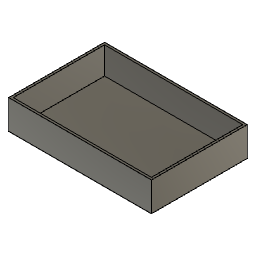
Container v1 (Autodesk Fusion 360 design; units mm, degrees)
Autodesk Fusion 360 part; units mm, degrees
sketch "Sketch1" plane through (0, 0, 0) normal (0, 0, 1) x (1, 0, 0)
  line L0 (63.38, 42.565) -> (-63.38, 42.565)
  line L1 (-63.38, 42.565) -> (-63.38, -42.565)
  line L2 (-63.38, -42.565) -> (63.38, -42.565)
  line L3 (63.38, -42.565) -> (63.38, 42.565)
  line L4 (63.38, 42.565) -> (-63.38, -42.565) construction
  line L5 (-63.38, 42.565) -> (63.38, -42.565) construction
  dimension "d1" = 126.76
  dimension "d2" = 85.13
  constraint horizontal L0
  constraint perpendicular L0 L1
  constraint parallel L0 L2
  constraint parallel L1 L3
  constraint coincident L4 origin
  constraint coincident L5 origin
  measures "d1" distance of L1.end L2.end
  measures "d2" distance of L0.end L1.end
extrude "Extrude1" add sketch "Sketch1" along normal blind 26
shell "Shell1" thickness 2 removed faces 1 at (21.1267, -14.1883, 26)
